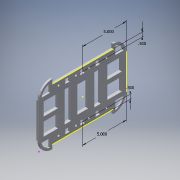
# Autodesk Inventor part: Frame 2.1
Saved by Autodesk Inventor 2018.2 (Build 222227000, 227)
## iProperties
Created: 2018-02-01
Part Number: Frame 2.1
Material: ABS Plastic
Document SubType Name: Modeling
Designer: MIABo
Density: 1.06 g/cm^3
Appearance: Smooth - White
Mass: 511.869 g
Surface Area: 864.604 cm^2
Volume: 482.895 cm^3
Author: MIABo
## iProperties of the stored document Frame 2_3DPrint.ipt
Created: 2018-03-02
Part Number: Frame 2_3DPrint
Material: Generic
Document SubType Name: Modeling
Designer: MIABo
Density: 1 g/cm^3
Appearance: Default
Author: MIABo
Autodesk Inventor part; units mm, degrees
ref_plane "YZ Plane" through (0, 0, 0) normal (1, 0, 0) x (0, 1, 0)
ref_plane "XZ Plane" through (0, 0, 0) normal (0, 1, 0) x (-1, 0, 0)
ref_plane "XY Plane" through (0, 0, 0) normal (0, 0, 1) x (1, 0, 0)
sketch "Sketch1" plane through (0, 0, 0) normal (1, 0, 0) x (0, 1, 0)
  line L0 (-76.2, 88.9) -> (-76.2, 88.9)
  line L1 (-50.8, 127) -> (50.8, 127)
  line L2 (50.8, -127) -> (-50.8, -127)
  line L3 (-76.2, -88.9) -> (-76.2, 88.9)
  arc A0 (88.9, 88.9) -> (50.8, 127) centre (50.8, 88.9) ccw
  line L4 (76.2, 88.9) -> (88.9, 88.9)
  arc A1 (-50.8, 127) -> (-88.9, 88.9) centre (-50.8, 88.9) ccw
  line L5 (-50.8, 88.9) -> (-88.9, 88.9)
  arc A2 (50.8, -127) -> (88.9, -88.9) centre (50.8, -88.9) ccw
  line L6 (76.2, -88.9) -> (88.9, -88.9)
  line L7 (76.2, 88.9) -> (76.2, -88.9)
  arc A3 (-88.9, -88.9) -> (-50.8, -127) centre (-50.8, -88.9) ccw
  line L8 (-76.2, -88.9) -> (-88.9, -88.9)
  point P0 (0, 0)
  point P1 (-76.2, 117.2981)
  point P2 (-76.2, -117.2981)
  dimension "d62" = 254
  dimension "d64" = 76.2
  dimension "d65" = 127
  dimension "d66" = 76.2
  dimension "d72" = 76.2
  dimension "d73" = 25.4
  dimension "d74" = 76.2
  dimension "d76" = 25.4
  dimension "d77" = 76.2
  dimension "d78" = 25.4
  constraints: 18 end point, 10 point on circle, 4 centre point, 4 horizontal, 4 tangent, 2 parallel, 2 perpendicular, 1 point on line
  measures "d62" distance between parallel lines of L2 L1
  measures "d64" distance from line of L3 point (0, 0)
  measures "d65" distance from line of L1 point (0, 0)
  measures "d66" diameter of A0
  measures "d72" diameter of A1
  measures "d73" distance from line of L3 L5.start
  measures "d74" diameter of A2
  measures "d76" distance from line of A2.centre L7
  measures "d77" diameter of A3
  measures "d78" distance from line of L3 A3.centre
extrude "Extrusion1" add sketch "Sketch1" along normal blind 5.08
sketch "Sketch3" plane through (5.08, 0, 0) normal (1, 0, 0) x (0, 0, -1)
  line L0 (88.9, 76.2) -> (-88.9, 76.2) projected
  line L1 (127, -50.8) -> (127, 50.8) projected
  line L2 (-88.9, -76.2) -> (88.9, -76.2) projected
  point P0 (0, 0)
  point P1 (0, -63.5)
  point P2 (0, 63.5)
  point P3 (0, 63.5)
  point P4 (127, 76.2)
  point P5 (127, -76.2)
  point P6 (-127, -76.2)
  dimension "d68" = 12.7
  dimension "d69" = 127
  dimension "d70" = 127
  dimension "d71" = 12.7
  constraints: 1 coincident
  measures "d68" distance from line of L0 point (0, 63.5)
  measures "d69" distance from line of L1 point (0, -63.5)
  measures "d70" distance from line of L1 point (0, 63.5)
  measures "d71" distance from line of L2 point (0, -63.5)
sketch "Sketch4" plane through (5.08, 0, 0) normal (1, 0, 0) x (0, 0, -1)
  line L0 (-127, 50.8) -> (-127, -50.8) projected
  line L1 (-127, 50.8) -> (127, 50.8)
  line L2 (127, 50.8) -> (127, -50.8)
  line L3 (127, -50.8) -> (-127, -50.8)
  line L4 (-127, -50.8) -> (-127, 50.8)
  point P0 (0, 0)
  point P1 (-88.9, 88.9)
  dimension "d79" = 101.6
  dimension "d80" = 38.1
  constraints: 8 end point, 2 parallel, 1 horizontal, 1 perpendicular, 1 point on line
  measures "d79" distance of L1.end L2.end
  measures "d80" distance from line of L1 point (-88.9, 88.9)
extrude "Extrusion2" add sketch "Sketch4" against normal blind 8.255
sketch "Sketch8" plane through (-3.175, 0, 0) normal (-1, 0, 0) x (0, 0, 1)
  line L0 (-114.3, -44.45) -> (-71.9667, -44.45)
  line L1 (-71.9667, -44.45) -> (-71.9667, -6.35)
  line L2 (-71.9667, -6.35) -> (-114.3, -6.35)
  line L3 (-114.3, -6.35) -> (-114.3, -44.45)
  line L4 (-127, -50.8) -> (127, -50.8) projected
  line L5 (127, 50.8) -> (-127, 50.8) projected
  line L6 (-127, 50.8) -> (-127, -50.8) projected
  line L7 (-127, -50.8) -> (-127, 50.8) projected
  line L8 (-127, 0) -> (127, 0)
  line L9 (127, 50.8) -> (127, -50.8) projected
  line L10 (-114.3, 44.45) -> (-71.9667, 44.45)
  line L11 (-71.9667, 44.45) -> (-71.9667, 6.35)
  line L12 (-71.9667, 6.35) -> (-114.3, 6.35)
  line L13 (-114.3, 6.35) -> (-114.3, 44.45)
  line L14 (-15.875, -38.1) -> (15.875, -38.1)
  line L15 (15.875, -38.1) -> (15.875, 38.1)
  line L16 (15.875, 38.1) -> (-15.875, 38.1)
  line L17 (-15.875, 38.1) -> (-15.875, -38.1)
  line L18 (-52.9167, 44.45) -> (-33.8667, 44.45)
  line L19 (-33.8667, 44.45) -> (-33.8667, -44.45)
  line L20 (-33.8667, -44.45) -> (-52.9167, -44.45)
  line L21 (-52.9167, -44.45) -> (-52.9167, 44.45)
  line L22 (-88.9, 76.2) -> (88.9, 76.2) projected
  line L23 (0, 76.2) -> (0, -76.2)
  line L24 (88.9, -76.2) -> (-88.9, -76.2) projected
  line L25 (114.3, -44.45) -> (71.9667, -44.45)
  line L26 (71.9667, -44.45) -> (71.9667, -6.35)
  line L27 (71.9667, -6.35) -> (114.3, -6.35)
  line L28 (114.3, -6.35) -> (114.3, -44.45)
  line L29 (114.3, 6.35) -> (114.3, 44.45)
  line L30 (71.9667, 6.35) -> (114.3, 6.35)
  line L31 (114.3, 44.45) -> (71.9667, 44.45)
  line L32 (71.9667, 44.45) -> (71.9667, 6.35)
  line L33 (52.9167, 44.45) -> (33.8667, 44.45)
  line L34 (33.8667, 44.45) -> (33.8667, -44.45)
  line L35 (33.8667, -44.45) -> (52.9167, -44.45)
  line L36 (52.9167, -44.45) -> (52.9167, 44.45)
  point P0 (0, 0)
  dimension "d95" = 6.35
  dimension "d96" = 101.6
  dimension "d97" = 44.45
  dimension "d98" = 12.7
  dimension "d99" = 42.3333
  dimension "d100" = 12.7
  dimension "d101" = 12.7
  dimension "d102" = 31.75
  dimension "d105" = 19.05
  dimension "d106" = 6.35
  dimension "d107" = 6.35
  dimension "d128" = 111.125
  dimension "d129" = 160.8667
  constraints: 60 end point, 16 symmetric about line, 6 parallel, 4 midpoint, 3 horizontal, 3 perpendicular
  measures "d95" distance between parallel lines of L4 L0
  measures "d96" distance between parallel lines of L5 L4
  measures "d97" distance between parallel lines of L4 L2
  measures "d98" distance between parallel lines of L6 L3
  measures "d99" distance between parallel lines of L3 L1
  measures "d100" distance between parallel lines of L14 L4
  measures "d101" distance between parallel lines of L5 L16
  measures "d102" distance of L15.end L16.end
  measures "d105" distance of L18.start L18.end
  measures "d106" distance between parallel lines of L5 L18
  measures "d107" distance between parallel lines of L4 L20
  measures "d128" distance between parallel lines of L9 L15
  measures "d129" distance between parallel lines of L9 L19
extrude "Extrusion5" cut sketch "Sketch8" against normal blind 25.4 contours L3 L2 L1 L0 | L23 L8 L15 L14 | L14 L17 L8 L23 | L21 L18 L19 L8 | L8 L19 L20 L21 | L23 L16 L15 L8 | L8 L17 L16 L23 | L36 L35 L34 L8 | L8 L34 L33 L36 | L10 L11 L12 L13 | L25 L26 L27 L28 | L30 L32 L31 L29
sketch "Sketch10" plane through (0, 0, 0) normal (-1, 0, 0) x (0, 0, 1)
  line L0 (-88.9, 76.2) -> (88.9, 76.2) projected
  line L1 (0, 76.2) -> (0, -76.2)
  line L2 (88.9, -76.2) -> (-88.9, -76.2) projected
  line L3 (88.9, 76.2) -> (88.9, 88.9) projected
  line L4 (127, 50.8) -> (127, -50.8) projected
  line L5 (127, 0) -> (-127, 0)
  line L6 (-127, 50.8) -> (-127, -50.8) projected
  point P0 (0, 0)
  point P1 (19.05, 63.5)
  point P2 (69.85, 63.5)
  point P3 (-19.05, 63.5)
  point P4 (-69.85, 63.5)
  point P5 (19.05, -63.5)
  point P6 (69.85, -63.5)
  point P7 (-19.05, -63.5)
  point P8 (-69.85, -63.5)
  dimension "d135" = 12.7
  dimension "d136" = 19.05
  dimension "d137" = 19.05
  dimension "d138" = 12.7
  constraints: 6 symmetric about line, 4 end point, 4 midpoint
  measures "d135" distance from line of L0 point (19.05, 63.5)
  measures "d136" distance from line of L1 point (19.05, 63.5)
  measures "d137" distance from line of point (69.85, 63.5) L3
  measures "d138" distance from line of L0 point (69.85, 63.5)
hole "Hole5" at (0, 63.5, 69.85) at (0, 63.5, 19.05) at (0, 63.5, -19.05) at (0, 63.5, -69.85) at (0, -63.5, -69.85) at (0, -63.5, -19.05) at (0, -63.5, 19.05) at (0, -63.5, 69.85) direction (1, 0, 0) diameter 6.35 end through all
sketch "Sketch11" plane through (0, 0, 0) normal (-1, 0, 0) x (0, 0, 1)
  line L0 (50.8, 69.85) -> (38.1, 69.85)
  line L1 (38.1, 69.85) -> (38.1, 57.15)
  line L2 (38.1, 57.15) -> (50.8, 57.15)
  line L3 (50.8, 57.15) -> (50.8, 69.85)
  line L4 (-88.9, 76.2) -> (88.9, 76.2) projected
  line L5 (127, 50.8) -> (-127, 50.8) projected
  line L6 (0, 76.2) -> (0, -76.2)
  line L7 (88.9, -76.2) -> (-88.9, -76.2) projected
  line L8 (0, 69.85) -> (6.35, 69.85)
  line L9 (6.35, 69.85) -> (6.35, 57.15)
  line L10 (6.35, 57.15) -> (0, 57.15)
  circle A0 centre (19.05, 63.5) radius 3.175 projected
  circle A1 centre (69.85, 63.5) radius 3.175 projected
  line L11 (-50.8, 69.85) -> (-38.1, 69.85)
  line L12 (-38.1, 69.85) -> (-38.1, 57.15)
  line L13 (-38.1, 57.15) -> (-50.8, 57.15)
  line L14 (-50.8, 57.15) -> (-50.8, 69.85)
  line L15 (0, 69.85) -> (-6.35, 69.85)
  line L16 (-6.35, 69.85) -> (-6.35, 57.15)
  line L17 (-6.35, 57.15) -> (0, 57.15)
  line L18 (120.0085, -57.15) -> (95.25, -57.15)
  line L19 (95.25, -57.15) -> (95.25, -81.9085)
  arc A2 (95.25, -81.9085) -> (120.0085, -57.15) centre (88.9, -50.8) ccw
  arc A3 (88.9, -88.9) -> (127, -50.8) centre (88.9, -50.8) ccw projected
  line L20 (-127, -50.8) -> (127, -50.8) projected
  line L21 (88.9, -88.9) -> (88.9, -76.2) projected
  line L22 (-120.0085, -57.15) -> (-95.25, -57.15)
  line L23 (-95.25, -57.15) -> (-95.25, -81.9085)
  arc A4 (-120.0085, -57.15) -> (-95.25, -81.9085) centre (-88.9, -50.8) ccw
  line L24 (127, 50.8) -> (127, -50.8) projected
  line L25 (127, 0) -> (-127, 0)
  line L26 (-127, -50.8) -> (-127, 50.8) projected
  line L27 (120.0085, 57.15) -> (95.25, 57.15)
  line L28 (95.25, 57.15) -> (95.25, 81.9085)
  arc A5 (120.0085, 57.15) -> (95.25, 81.9085) centre (88.9, 50.8) ccw
  arc A6 (-95.25, 81.9085) -> (-120.0085, 57.15) centre (-88.9, 50.8) ccw
  line L29 (-120.0085, 57.15) -> (-95.25, 57.15)
  line L30 (-95.25, 57.15) -> (-95.25, 81.9085)
  line L31 (50.8, -69.85) -> (38.1, -69.85)
  line L32 (38.1, -69.85) -> (38.1, -57.15)
  line L33 (38.1, -57.15) -> (50.8, -57.15)
  line L34 (50.8, -57.15) -> (50.8, -69.85)
  line L35 (0, -69.85) -> (6.35, -69.85)
  line L36 (6.35, -69.85) -> (6.35, -57.15)
  line L37 (6.35, -57.15) -> (0, -57.15)
  line L38 (-50.8, -57.15) -> (-50.8, -69.85)
  line L39 (-38.1, -57.15) -> (-50.8, -57.15)
  line L40 (-50.8, -69.85) -> (-38.1, -69.85)
  line L41 (-38.1, -69.85) -> (-38.1, -57.15)
  line L42 (-6.35, -69.85) -> (-6.35, -57.15)
  line L43 (-6.35, -57.15) -> (0, -57.15)
  line L44 (0, -69.85) -> (-6.35, -69.85)
  point P0 (0, 0)
  dimension "d146" = 6.35
  dimension "d147" = 6.35
  dimension "d148" = 12.7
  dimension "d149" = 6.35
  dimension "d152" = 19.05
  dimension "d153" = 50.8
  dimension "d154" = 6.35
  dimension "d155" = 6.35
  dimension "d156" = 6.35
  dimension "d159" = 31.75
  constraints: 76 end point, 32 symmetric about line, 8 point on circle, 5 perpendicular, 4 centre point, 4 midpoint, 2 collinear, 2 horizontal, 2 parallel, 2 point on line, 1 concentric, 3 other
  measures "d146" distance between parallel lines of L4 L0
  measures "d147" distance between parallel lines of L5 L2
  measures "d148" distance of L0.start L0.end
  measures "d149" distance of L8.start L8.end
  measures "d152" distance from line of L1 A0.centre
  measures "d153" distance of A1.centre A0.centre
  measures "d154" distance between parallel lines of L18 L20
  measures "d155" radial gap between concentric circles of A3 A2
  measures "d156" distance between parallel lines of L21 L19
  measures "d159" distance between parallel lines of L9 L1
extrude "Extrusion6" cut sketch "Sketch11" against normal blind 25.4 contours L3 L2 L1 L0 | L17 L16 L15 L6 | L6 L8 L9 L10 | L37 L36 L35 L6 | L6 L44 L42 L43 | L11 L12 L13 L14 | A2 L19 L18 | L22 L23 A4 | L27 L28 A5 | L30 L29 A6 | L31 L32 L33 L34 | L39 L41 L40 L38
body "Solid1"
